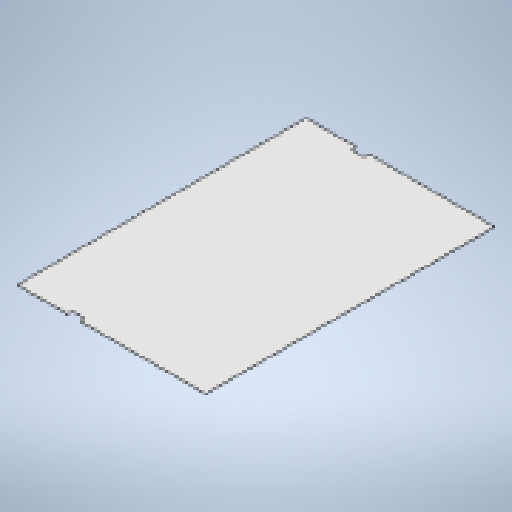
# Autodesk Inventor part: GnG frame 1.1 floor sheet 3
Saved by Autodesk Inventor 2025.3 (Build 293356030, 356C)
## iProperties
Created: 2025-10-28
Part Number: GnG frame 1.1 floor sheet 3
Material: Stainless Steel
Document SubType Name: Sheet Metal
Designer: admin
Mass: 280.619 g
Surface Area: 364.406 cm^2
Volume: 35.0774 cm^3
Density: 8 g/cm^3
Sheet Metal Rule: AISI304 3mm Die 32
Sheet Metal Width: 1500,000 mm
Sheet Metal Length: 2300,000 mm
Sheet Metal Area: 3450000,000 mm^2
Appearance: Default
Stock Number: 1.3
Flat Pattern Width: 150 cm
Flat Pattern Length: 230 cm
Flat Pattern Area: 34500 cm^2
Author: admin
Autodesk Inventor part; units mm, degrees
ref_plane "YZ Plane" through (0, 0, 0) normal (1, 0, 0) x (0, 1, 0)
ref_plane "XZ Plane" through (0, 0, 0) normal (0, 1, 0) x (-1, 0, 0)
ref_plane "XY Plane" through (0, 0, 0) normal (0, 0, 1) x (1, 0, 0)
sketch "Sketch1" plane through (0, 0, 0) normal (0, 0, 1) x (1, 0, 0)
  line L0 (0, 0) -> (-1500, 0)
  line L1 (-1500, 0) -> (-1500, -2300)
  line L2 (-1500, -2300) -> (0, -2300)
  line L3 (0, -2300) -> (0, 0)
  line L4 (0, 0) -> (-40, 0)
  line L5 (-40, 0) -> (-40, -40)
  line L6 (-40, -40) -> (0, -40)
  line L7 (0, -40) -> (0, 0)
  line L8 (0, -2300) -> (-40, -2300)
  line L9 (-40, -2300) -> (-40, -2260)
  line L10 (-40, -2260) -> (0, -2260)
  line L11 (0, -2260) -> (0, -2300)
  line L12 (-1500, 0) -> (-1460, 0)
  line L13 (-1460, 0) -> (-1460, -40)
  line L14 (-1460, -40) -> (-1500, -40)
  line L15 (-1500, -40) -> (-1500, 0)
  line L16 (-1500, -2300) -> (-1460, -2300)
  line L17 (-1460, -2300) -> (-1460, -2260)
  line L18 (-1460, -2260) -> (-1500, -2260)
  line L19 (-1500, -2260) -> (-1500, -2300)
  line L20 (-960, -2300) -> (-860, -2300)
  line L21 (-860, -2300) -> (-860, -2260)
  line L22 (-860, -2260) -> (-960, -2260)
  line L23 (-960, -2260) -> (-960, -2300)
  line L24 (-960, 0) -> (-860, 0)
  line L25 (-860, 0) -> (-860, -40)
  line L26 (-860, -40) -> (-960, -40)
  line L27 (-960, -40) -> (-960, 0)
  point P0 (0, -40)
  point P1 (-40, 0)
  point P2 (0, -2260)
  point P3 (-860, 0)
  dimension "d22" = 1500
  dimension "d23" = 2300
  dimension "d24" = 40
  dimension "d25" = 40
  dimension "d28" = 100
  dimension "d29" = 820
  measures "d22" distance of L2.end L1.end
  measures "d23" distance of L1.end L0.end
  measures "d24" distance of L6.end L5.end
  measures "d25" distance of L5.end L4.end
  measures "d28" distance of L25.end L26.end
  measures "d29" distance between parallel lines of L5 L25
extrude "Plate1" add sketch "Sketch1" along normal blind 3 contours L3 L6 L5 L0 | L5 L6 L3 L10 L9 L2 L21 L22 L23 L17 L18 L1 L14 L13 L0 L27 L26 L25 | L3 L2 L9 L10 | L13 L14 L1 L0 | L18 L17 L2 L1
sketch "Sketch6" plane through (0, 0, 3) normal (0, 0, 1) x (1, 0, 0)
  line L0 (-1395, 0) -> (-1390, 0)
  line L1 (-1375, -5) -> (-1375, 0)
  line L2 (-1375, 0) -> (-1370, 0)
  line L3 (-1370, 0) -> (-1370, -5)
  line L4 (-1370, 0) -> (-1365, 0) construction
  line L5 (-1365, 0) -> (-1363.6916, -4.1277)
  arc A0 (-1363.6916, -4.1277) -> (-1361.3084, -4.1277) centre (-1362.5, -3.75) ccw
  line L6 (-1365, 0) -> (-1360, 0)
  line L7 (-1360, 0) -> (-1355, 0) construction
  line L8 (-1355, -5) -> (-1355, 0)
  line L9 (-1350, -5) -> (-1355, -5)
  line L10 (-1350, 0) -> (-1350, -5)
  line L11 (-1355, 0) -> (-1350, 0)
  line L12 (-1350, -2.5) -> (-1345, -2.5) construction
  line L13 (-1361.3084, -4.1277) -> (-1360, 0)
  line L14 (-1390, 0) -> (-1390, -5)
  line L15 (-1390, -5) -> (-1395, -5)
  line L16 (-1395, -5) -> (-1395, 0)
  line L17 (-1370, -5) -> (-1375, -5)
  line L18 (-1380, 0) -> (-1380, -5)
  line L19 (-1380, -5) -> (-1385, -5)
  line L20 (-1385, -5) -> (-1385, 0)
  line L21 (-1385, 0) -> (-1380, 0)
  line L22 (-1380, -2.5) -> (-1375, -2.5) construction
  line L23 (-1390, -2.5) -> (-1385, -2.5) construction
  line L24 (-1345, -5) -> (-1345, 0)
  line L25 (-1340, 0) -> (-1340, -5)
  line L26 (-1340, -5) -> (-1345, -5)
  line L27 (-1345, 0) -> (-1340, 0)
  line L28 (-1340, -2.5) -> (-1335, -2.5) construction
  line L29 (-1335, -5) -> (-1335, 0)
  line L30 (-1335, 0) -> (-1330, 0)
  line L31 (-1330, -5) -> (-1335, -5)
  arc A1 (-1402.5, 0) -> (-1397.5, 0) centre (-1400, 0) ccw
  line L32 (-1330, 0) -> (-1330, -5)
  line L33 (-1500, 0) -> (-960, 0) projected
  line L34 (-1500, -2300) -> (-1500, 0) projected
  point P0 (0, 0)
  point P1 (-1362.5, 0)
  dimension "d38" = 5
  dimension "d39" = 5
  dimension "d40" = 1.25
  dimension "d41" = 5
  dimension "d42" = 5
  dimension "d43" = 5
  dimension "d44" = 5
  dimension "d45" = 5
  dimension "d46" = 100
  constraints: 66 end point, 12 parallel, 11 horizontal, 10 equal length, 9 midpoint, 6 perpendicular, 5 collinear, 4 point on circle, 4 point on line, 3 tangent, 2 centre point, 1 vertical alignment
  measures "d38" distance of L14.end L16.start
  measures "d39" distance of L16.start L0.start
  measures "d40" radius of A0
  measures "d41" distance of L5.start L6.end
  measures "d42" distance of L10.end L8.start
  measures "d43" distance of L8.start L7.end
  measures "d44" diameter of A1
  measures "d45" distance of A1.centre L0.start
  measures "d46" distance from line of L34 A1.centre
extrude "Cut1" cut sketch "Sketch6" against normal blind 3 contours L0 L14 L15 L16 | L1 L2 L3 L17 | L18 L19 L20 L21 | L33 A1
equation "\"d24\" = d25"
equation "\"d40\" = 0.25 * d38"
equation "\"d47\" = Thickness"
equation "\"d2\" = Thickness"
equation "\"BendReliefWidth\" = Thickness"
equation "\"BendReliefDepth\" = 0.5 * Thickness"
equation "\"CornerReliefSize\" = 4 * Thickness"
equation "\"MinimumRemnant\" = 2 * Thickness"
equation "\"TransitionRadius\" = BendRadius"
equation "\"JacobiRadiusSize\" = BendRadius"
equation "\"GapSize\" = Thickness"
equation "\"Thickness\" = 3"
equation "\"BendRadius\" = 5"
body "Solid1"
